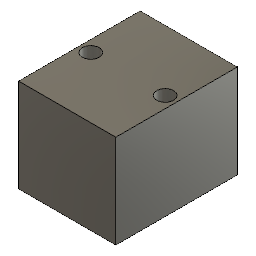
LEDFitTest (Autodesk Fusion 360 design; units mm, degrees)
Autodesk Fusion 360 part; units mm, degrees
sketch "Sketch1" plane through (0, 0, 0) normal (1, 0, 0) x (0, 0, -1)
sketch "Sketch2" plane through (0, 0, 0) normal (0, 1, 0) x (1, 0, 0)
  line L0 (0, 0) -> (2.75, 0)
  line L1 (0, 0) -> (-2.75, 0)
  line L2 (0, 0) -> (5.2, 0)
  line L3 (0, 0) -> (-5.2, 0)
  circle A0 centre (-3.975, 0) radius 1.225
  circle A1 centre (3.975, 0) radius 1.225
  line L4 (5.2, 6.5) -> (-5.2, 6.5)
  line L5 (-5.2, 6.5) -> (-5.2, -6.5)
  line L6 (-5.2, -6.5) -> (5.2, -6.5)
  line L7 (5.2, -6.5) -> (5.2, 6.5)
  line L8 (5.2, 6.5) -> (-5.2, -6.5) construction
  line L9 (-5.2, 6.5) -> (5.2, -6.5) construction
  circle A2 centre (-3.975, 0) radius 0.9
  circle A3 centre (3.975, 0) radius 0.9
  dimension "d1" = 2.75
  dimension "d2" = 2.75
  dimension "d3" = 5.2
  dimension "d4" = 13
  dimension "d7" = 1.8
  dimension "d8" = 1.8
  dimension "d10" = 2.45
  measures "d1" distance of L0.start
  measures "d2" distance of L0.start
  measures "d3" distance of L0.start
  measures "d7" diameter of A2
  measures "d8" diameter of A3
  measures "d10" diameter of A0
extrude "Extrude1" add sketch "Sketch2" along normal blind 10 contours L0 L1 L2 L3 A0 A1 L4 L5 L7 | L0 L1 L2 L3 A0 A1 L5 L6 L7 | L2 A1 A3 | L2 A1 A3 | L3 A0 A2 | L3 A0 A2
fillet "Fillet1" [rolled back] radius 1.202
equation "d1 = ( 5.5 / 2 ) * 1 mm"
equation "d2 = ( 5.5 / 2 ) * 1 mm"
equation "d3 = ( 10.4 / 2 ) * 1 mm"
